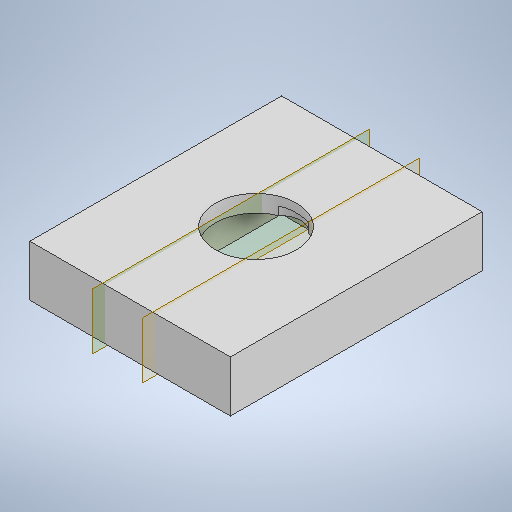
# Autodesk Inventor part: sensor bulet + magnet tes 1
Saved by Autodesk Inventor 2025.3 (Build 293356000, 356)
## iProperties
Created: 2026-02-16
Part Number: sensor bulet + magnet tes 1
Material: Generic
Document SubType Name: Modeling
Designer: Maulana
Density: 1 g/cm^3
Appearance: Default
Author: Maulana
Autodesk Inventor part; units mm, degrees
sketch "Sketch1" plane through (0, 0, 0) normal (0, 1, 0) x (-1, 0, 0)
  line L0 (-11.75, 14.75) -> (11.75, 14.75)
  line L1 (11.75, 14.75) -> (11.75, -14.75)
  line L2 (11.75, -14.75) -> (-11.75, -14.75)
  line L3 (-11.75, -14.75) -> (-11.75, 14.75)
  line L4 (-11.75, 14.75) -> (11.75, -14.75) construction
  line L5 (11.75, 14.75) -> (-11.75, -14.75) construction
  line L6 (-5.75, 8.75) -> (5.75, 8.75)
  line L7 (5.75, 8.75) -> (5.75, -8.75)
  line L8 (5.75, -8.75) -> (-5.75, -8.75)
  line L9 (-5.75, -8.75) -> (-5.75, 8.75)
  line L10 (-5.75, 8.75) -> (5.75, -8.75) construction
  line L11 (5.75, 8.75) -> (-5.75, -8.75) construction
  point P0 (0, 0)
  dimension "d0" = 23.5
  dimension "d1" = 29.5
  dimension "d2" = 11.5
  dimension "d3" = 17.5
  constraints: 24 end point, 4 midpoint, 4 parallel, 2 horizontal, 2 perpendicular
  measures "d0" distance of L1.end L2.end
  measures "d1" distance of L0.end L1.end
  measures "d2" distance of L7.end L8.end
  measures "d3" distance of L6.end L7.end
extrude "Extrusion1" add sketch "Sketch1" along normal blind 6
sketch "Sketch2" plane through (0, 6, 0) normal (0, 1, 0) x (1, 0, 0)
  circle A0 centre (0, 0) radius 4.75
  line L0 (5.75, -8.75) -> (-5.75, -8.75) projected
  line L1 (-5.75, -8.75) -> (5.75, -8.75)
  line L2 (5.75, -8.75) -> (5.75, 8.75)
  line L3 (5.75, 8.75) -> (-5.75, 8.75)
  line L4 (-5.75, 8.75) -> (-5.75, -8.75)
  dimension "d6" = 9.5
  constraints: 8 end point, 2 parallel, 1 centre point, 1 coincident, 1 horizontal, 1 perpendicular
  measures "d6" diameter of A0
extrude "Extrusion2" add sketch "Sketch2" against normal blind 2
sketch "Sketch4" plane through (0, 4, 0) normal (0, -1, 0) x (1, 0, 0)
  line L0 (-5.75, 8.75) -> (5.75, 8.75) projected
  line L1 (-5.75, -8.75) -> (-5.75, 8.75) projected
  line L2 (5.75, 8.75) -> (-5.75, 8.75)
  line L3 (-5.75, 8.75) -> (-5.75, 6.25)
  line L4 (-5.75, 6.25) -> (5.75, 6.25)
  line L5 (5.75, 6.25) -> (5.75, 8.75)
  point P0 (0, 0)
  dimension "d9" = 2.5
  constraints: 8 end point, 2 parallel, 1 horizontal, 1 perpendicular, 1 point on line
  measures "d9" distance of L3.end L2.end
sketch "Sketch5" plane through (0, 0, 0) normal (0, -1, 0) x (1, 0, 0)
  line L0 (-5.75, -8.75) -> (5.75, -8.75) projected
  line L1 (0, -8.75) -> (0, -11.75)
  line L2 (11.75, -14.75) -> (-11.75, -14.75) projected
  circle A0 centre (0, -11.75) radius 2.25
  point P0 (0, 0)
  dimension "d10" = 3
  dimension "d11" = 4.5
  constraints: 2 end point, 1 centre point, 1 coincident, 1 midpoint, 1 perpendicular
  measures "d10" distance of L1.start L1.end
  measures "d11" diameter of A0
extrude "Extrusion3" cut sketch "Sketch5" against normal blind 5
ref_plane "Work Plane1" through (0, 0, 14.75) normal (1, 0, 0) x (0, 0, -1)
ref_plane "Work Plane2" through (11.75, 0, 0) normal (0, 0, -1) x (-1, 0, 0)
ref_plane "Work Plane3" through (-5.875, 0, -14.75) normal (-1, 0, 0) x (0, 0, 1)
ref_plane "Work Plane4" through (5.875, 0, 14.75) normal (1, 0, 0) x (0, 0, -1)
ref_plane "Work Plane6" through (4.4063, 0, 14.75) normal (1, 0, 0) x (0, 0, -1)
ref_plane "Work Plane5" through (-2.9375, 0, -14.75) normal (-1, 0, 0) x (0, 0, 1)
ref_plane "Work Plane8" through (-4.4062, 0, -14.75) normal (-1, 0, 0) x (0, 0, 1)
ref_plane "Work Plane7" through (2.9375, 0, 14.75) normal (1, 0, 0) x (0, 0, -1)
mirror "Mirror2" about plane through (11.75, 0, 0) normal (0, 0, -1) of "Extrusion3"
mirror "Mirror3" about plane through (4.4063, 0, 14.75) normal (1, 0, 0) of "Extrusion3", "Mirror2"
mirror "Mirror4" about plane through (-4.4062, 0, -14.75) normal (-1, 0, 0) of "Extrusion3", "Mirror2"
ref_plane "Work Plane9" through (11.75, 0, -7.375) normal (0, 0, -1) x (-1, 0, 0)
ref_plane "Work Plane10" through (-11.75, 0, 7.375) normal (0, 0, 1) x (1, 0, 0)
mirror "Mirror5" about plane through (-11.75, 0, 7.375) normal (0, 0, 1) of "Extrusion3", "Mirror2", "Mirror4", "Mirror3"
mirror "Mirror6" about plane through (11.75, 0, -7.375) normal (0, 0, -1) of "Extrusion3", "Mirror2", "Mirror4", "Mirror3"
extrude "Extrusion4" add sketch "Sketch4" along normal blind 1
sketch "Sketch7" plane through (11.75, 0, -14.75) normal (0, 0, -1) x (-1, 0, 0)
  line L0 (23.5, 0) -> (23.5, 6) projected
  line L1 (23.5, 0) -> (17.5, 0)
  line L2 (17.5, 0) -> (17.5, 4)
  line L3 (17.5, 4) -> (23.5, 4)
  line L4 (23.5, 4) -> (23.5, 0)
  line L5 (0, 0) -> (0, 6) projected
  line L6 (0, 0) -> (6, 0)
  line L7 (6, 0) -> (6, 4)
  line L8 (6, 4) -> (0, 4)
  line L9 (0, 4) -> (0, 0)
  point P0 (11.75, 0)
  dimension "d16" = 6
  dimension "d17" = 4
  dimension "d18" = 6
  dimension "d19" = 4
  constraints: 16 end point, 4 parallel, 2 horizontal, 2 perpendicular
  measures "d16" distance of L2.end L3.end
  measures "d17" distance of L1.end L2.end
  measures "d18" distance of L8.end L7.end
  measures "d19" distance of L7.end L6.end
extrude "Extrusion5" add sketch "Sketch7" against normal blind 29.5
sketch "Sketch8" plane through (-11.75, 0, -14.75) normal (-1, 0, 0) x (0, 0, 1)
  line L0 (29.5, 0) -> (29.5, 6) projected
  line L1 (29.5, 0) -> (23.5, 0)
  line L2 (23.5, 0) -> (23.5, 4)
  line L3 (23.5, 4) -> (29.5, 4)
  line L4 (29.5, 4) -> (29.5, 0)
  line L5 (0, 0) -> (0, 6) projected
  line L6 (0, 0) -> (6, 0)
  line L7 (6, 0) -> (6, 4)
  line L8 (6, 4) -> (0, 4)
  line L9 (0, 4) -> (0, 0)
  point P0 (14.75, 0)
  dimension "d22" = 6
  dimension "d23" = 4
  dimension "d24" = 6
  dimension "d25" = 4
  constraints: 16 end point, 4 parallel, 2 horizontal, 2 perpendicular
  measures "d22" distance of L2.end L3.end
  measures "d23" distance of L1.end L2.end
  measures "d24" distance of L8.end L7.end
  measures "d25" distance of L7.end L6.end
extrude "Extrusion6" add sketch "Sketch8" against normal blind 23.5
body "Solid1"
